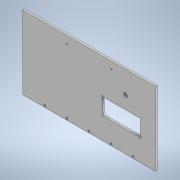
# Autodesk Inventor part: sheetmetalright2.0
Saved by Autodesk Inventor 2020.2 (Build 242310000, 310)
## iProperties
Created: 2020-02-06
Part Number: sheetmetalright2.0
Material: Generic
Document SubType Name: Sheet Metal
Designer: ColinP
Density: 1 g/cm^3
Sheet Metal Rule: Default
Appearance: Default
Author: ColinP
Autodesk Inventor part; units mm, degrees
ref_plane "YZ Plane" through (0, 0, 0) normal (1, 0, 0) x (0, 1, 0)
ref_plane "XZ Plane" through (0, 0, 0) normal (0, 1, 0) x (-1, 0, 0)
ref_plane "XY Plane" through (0, 0, 0) normal (0, 0, 1) x (1, 0, 0)
sketch "Sketch1" plane through (0, 0, 0) normal (0, 0, 1) x (1, 0, 0)
  line L0 (114.3, 63.5) -> (-114.3, 63.5)
  line L1 (-114.3, 63.5) -> (-114.3, -63.5)
  line L2 (-114.3, -63.5) -> (114.3, -63.5)
  line L3 (114.3, -63.5) -> (114.3, 63.5)
  point P0 (0, 0)
  dimension "d0" = 228.6
  dimension "d1" = 127
  measures "d0" distance of L2.end L1.end
  measures "d1" distance of L1.end L0.end
extrude "Plate1" add sketch "Sketch1" along normal blind 3.048
sketch "Sketch2" plane through (0, 0, 3.048) normal (0, 0, 1) x (1, 0, 0)
  line L0 (-114.3, -63.5) -> (114.3, -63.5) projected
  line L1 (114.3, -63.5) -> (114.3, -60.325)
  line L2 (114.3, -63.5) -> (114.3, 63.5) projected
  line L3 (114.3, -60.325) -> (76.2, -60.325)
  line L4 (76.2, -60.325) -> (38.1, -60.325)
  line L5 (38.1, -60.325) -> (0, -60.325)
  line L6 (0, -60.325) -> (-38.1, -60.325)
  line L7 (-38.1, -60.325) -> (-76.2, -60.325)
  line L8 (-76.2, -60.325) -> (-114.3, -60.325)
  line L9 (-114.3, 63.5) -> (-114.3, -63.5) projected
  point P0 (0, 0)
  dimension "d3" = 3.175
  dimension "d4" = 38.1
  dimension "d5" = 38.1
  dimension "d6" = 38.1
  dimension "d7" = 38.1
  constraints: 14 end point, 6 point on line, 1 horizontal, 1 perpendicular
  measures "d3" distance of L0.end L1.end
  measures "d4" distance of L1.end L3.end
  measures "d5" distance of L3.end L4.end
  measures "d6" distance of L5.end L6.end
  measures "d7" distance of L6.end L7.end
hole "Hole1" at (-76.2, -60.325, 3.048) at (-38.1, -60.325, 3.048) at (0, -60.325, 3.048) at (38.1, -60.325, 3.048) at (76.2, -60.325, 3.048) direction (0, 0, -1) diameter 3.2766 depth 3.048 clearance for "Hex Machine Screw" size "#4" standard "Ansi Unified Screw Threads"
sketch "Sketch3" plane through (0, 0, 3.048) normal (0, 0, 1) x (1, 0, 0)
  line L0 (114.3, -63.5) -> (114.3, -25.4)
  line L1 (114.3, -63.5) -> (114.3, 63.5) projected
  line L2 (114.3, -25.4) -> (88.9, -25.4)
  line L3 (88.9, -25.4) -> (22.86, -25.4)
  line L4 (22.86, -25.4) -> (22.86, 2.54)
  line L5 (22.86, 2.54) -> (88.9, 2.54)
  line L6 (88.9, 2.54) -> (88.9, -25.4)
  point P0 (0, 0)
  dimension "d15" = 38.1
  dimension "d16" = 25.4
  dimension "d17" = 66.04
  dimension "d18" = 27.94
  constraints: 12 end point, 4 perpendicular, 1 horizontal, 1 point on line
  measures "d15" distance of L0.start L0.end
  measures "d16" distance of L0.end L2.end
  measures "d17" distance of L2.end L3.end
  measures "d18" distance of L3.end L4.end
extrude "Cut1" cut sketch "Sketch3" against normal blind 3.048
sketch "Sketch4" plane through (0, 0, 3.048) normal (0, 0, 1) x (1, 0, 0)
  line L0 (114.3, 63.5) -> (-114.3, 63.5) projected
  line L1 (-114.3, 63.5) -> (-114.3, 50.8)
  line L2 (-114.3, -63.5) -> (-114.3, 63.5) projected
  line L3 (-114.3, 50.8) -> (-38.1, 50.8)
  line L4 (-38.1, 50.8) -> (38.1, 50.8)
  line L5 (38.1, 50.8) -> (114.3, 50.8)
  point P0 (0, 0)
  dimension "d21" = 12.7
  dimension "d22" = 76.2
  dimension "d23" = 76.2
  dimension "d24" = 76.2
  constraints: 8 end point, 3 point on line, 1 perpendicular
  measures "d21" distance of L0.end L1.end
  measures "d22" distance of L1.end L3.end
  measures "d23" distance of L3.end L4.end
  measures "d24" distance of L4.end L5.end
hole "Hole2" at (-38.1, 50.8, 3.048) at (38.1, 50.8, 3.048) direction (0, 0, -1) diameter 2.1565 end through all thread size "4-40 UNC" class "2B" standard "ANSI Unified Screw Threads"
sketch "Sketch5" plane through (0, 0, 3.048) normal (0, 0, 1) x (1, 0, 0)
  circle A0 centre (-38.1, 50.8) radius 1.0782 projected
  circle A1 centre (38.1, 50.8) radius 1.0782 projected
  line L0 (22.86, 2.54) -> (88.9, 2.54) projected
  line L1 (88.9, 2.54) -> (88.9, -25.4) projected
  line L2 (88.9, -25.4) -> (22.86, -25.4) projected
  line L3 (22.86, -25.4) -> (22.86, 2.54) projected
  circle A2 centre (38.1, -60.325) radius 1.6383 projected
  circle A3 centre (-38.1, -60.325) radius 1.6383 projected
  circle A4 centre (-76.2, -60.325) radius 1.6383 projected
  circle A5 centre (0, -60.325) radius 1.6383 projected
  circle A6 centre (76.2, -60.325) radius 1.6383 projected
  line L4 (114.3, 63.5) -> (114.3, -63.5) projected
  line L5 (-114.3, 63.5) -> (114.3, 63.5) projected
  line L6 (-114.3, -63.5) -> (-114.3, 63.5) projected
  line L7 (114.3, -63.5) -> (-114.3, -63.5) projected
  point P0 (0, 0)
hole "Hole3" at (22.86, 2.54, 3.048) at (88.9, 2.54, 3.048) at (88.9, -25.4, 3.048) at (22.86, -25.4, 3.048) direction (0, 0, -1) diameter 2.794 depth 3.048 clearance for "Flat Head Machine Screw (82)" size "#3" standard "Ansi Unified Screw Threads"
sketch "Sketch6" plane through (0, 0, 3.048) normal (0, 0, 1) x (1, 0, 0)
  line L0 (114.3, -63.5) -> (-114.3, -63.5) projected
  line L1 (114.3, -63.5) -> (63.5, -63.5)
  line L2 (63.5, -63.5) -> (63.5, 25.4)
  point P0 (0, 0)
  dimension "d39" = 50.8
  dimension "d40" = 88.9
  constraints: 4 end point, 1 perpendicular, 1 point on line
  measures "d39" distance of L0.start L1.end
  measures "d40" distance of L1.end L2.end
hole "Hole4" at (63.5, 25.4, 3.048) direction (0, 0, -1) diameter 6.7564 depth 3.048 clearance for "Flat Head Machine Screw (82)" size "1/4" standard "Ansi Unified Screw Threads"
equation "\"d13\" = Thickness"
equation "\"d19\" = Thickness"
equation "\"d37\" = Thickness"
equation "\"d46\" = Thickness"
equation "\"d2\" = Thickness"
equation "\"BendRadius\" = Thickness"
equation "\"BendReliefWidth\" = Thickness"
equation "\"BendReliefDepth\" = 0.5 * Thickness"
equation "\"CornerReliefSize\" = 4 * Thickness"
equation "\"MinimumRemnant\" = 2 * Thickness"
equation "\"TransitionRadius\" = BendRadius"
equation "\"JacobiRadiusSize\" = BendRadius"
equation "\"GapSize\" = Thickness"
equation "\"Thickness\" = 3.048"
body "Solid1"
